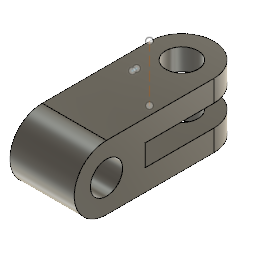
hinge1 (Autodesk Fusion 360 design; units mm, degrees)
Autodesk Fusion 360 part; units mm, degrees
note: some values were not read from the file. Set by a fixed rule: which sketch regions a step uses.
sketch "Sketch1" plane through (0, 0, 0) normal (1, 0, 0) x (0, 1, 0)
  line L0 (0, 0) -> (250, 0)
  line L1 (250, 0) -> (250, 150)
  line L2 (250, 150) -> (0, 150)
  line L3 (0, 150) -> (0, 0)
  circle A0 centre (0, 75) radius 75
  dimension "d1" = 250
  dimension "d2" = 150
  constraint coincident L0.start L3.end
  constraint horizontal L0
  constraint perpendicular L0 L1
  constraint perpendicular L1 L2
  constraint perpendicular L0 L3
  constraint coincident L2.end A0
  constraint tangent L2 A0
  constraint coincident L0.start A0
  measures "d1" distance of L0.start L0.end
  measures "d2" distance of L0.end L1.end
sketch "Sketch2" plane through (0, 0, 0) normal (1, 0, 0) x (0, 1, 0)
extrude "Extrude1" add sketch "Sketch1" along normal blind 150
sketch "Sketch3" plane through (0, 0, 0) normal (-1, 0, 0) x (0, -1, 0)
  line L0 (0, 150) -> (-250, 150)
  line L1 (-250, 150) -> (-250, 0)
  line L2 (-250, 0) -> (0, 0)
  arc A0 (0, 0) -> (0, 150) centre (0, 75) ccw
  line L3 (0, 150) -> (0, 0)
  circle A1 centre (0, 75) radius 37.5
  dimension "d5" = 75
  constraint coincident L0.start A0.end
  constraint coincident L2.end A0.start
  constraint concentric A0 A1
  measures "d5" diameter of A1
extrude "Extrude2" cut sketch "Sketch3" against normal blind 150 contours L3 A1 | L3 A1
sketch "Sketch4" plane through (150, 0, 0) normal (1, 0, 0) x (0, 1, 0)
  circle A0 centre (0, 75) radius 37.5
  line L0 (250, 150) -> (0, 150)
  arc A1 (0, 150) -> (0, 0) centre (0, 75) ccw
  line L1 (0, 0) -> (250, 0)
  line L2 (250, 0) -> (250, 150)
  line L3 (250, 150) -> (250, 0) construction
  line L4 (250, 75) -> (90, 75) construction
  line L5 (90, 75) -> (90, 100)
  line L6 (90, 75) -> (90, 50)
  line L7 (90, 100) -> (250, 100)
  line L8 (250, 50) -> (90, 50)
  dimension "d8" = 25
  dimension "d9" = 25
  constraint coincident L0.start L2.end
  constraint coincident L1.end L2.start
  constraint midpoint L2 L4.start
  constraint perpendicular L2 L4
  constraint perpendicular L0 L5
  constraint perpendicular L4 L6
  constraint coincident L2 L7.end
  constraint perpendicular L2 L7
  constraint coincident L2 L8.start
  constraint perpendicular L6 L8
  measures "d8" distance of L4.end L5.end
  measures "d9" distance of L4.end L6.end
extrude "Extrude3" cut sketch "Sketch4" against normal blind 150 contours L2 L5 L6 L7 L8
sketch "Sketch5" plane through (0, 0, 0) normal (0, 0, -1) x (1, 0, 0)
  line L0 (0, 0) -> (0, -250)
  line L1 (0, -250) -> (150, -250)
  line L2 (150, -250) -> (150, 0)
  line L3 (150, 0) -> (0, 0)
  line L4 (0, -250) -> (150, -250) construction
  circle A0 centre (75, -250) radius 75
  dimension "d12" = 150
  constraint coincident L0.end L1.start
  constraint coincident L1.end L2.start
  constraint midpoint L1 A0.centre
  measures "d12" diameter of A0
extrude "Extrude4" add sketch "Sketch5" against normal blind 50 contours L1 A0 picked at (76.8683, -274.9301)
sketch "Sketch6" plane through (0, 0, 0) normal (1, 0, 0) x (0, 1, 0)
  line L0 (220, 110) -> (210, 110)
  line L1 (250, 150) -> (250, 20) construction
  constraint horizontal L0
  constraint vertical L1
sketch "Sketch7" plane through (0, 0, 150) normal (0, 0, 1) x (-1, 0, 0)
  line L0 (0, -250) -> (0, 0)
  line L1 (0, 0) -> (-150, 0)
  line L2 (-150, 0) -> (-150, -250)
  line L3 (-150, -250) -> (0, -250)
  circle A0 centre (-75, -250) radius 75
  dimension "d15" = 150
  constraint midpoint L3 A0.centre
  measures "d15" diameter of A0
extrude "Extrude5" add sketch "Sketch7" against normal blind 50 contours L3 A0 picked at (-76.8683, -274.9301)
sketch "Sketch8" plane through (0, 0, 150) normal (0, 0, 1) x (-1, 0, 0)
  line L0 (0, -250) -> (0, 0)
  line L1 (0, 0) -> (-150, 0)
  line L2 (-150, 0) -> (-150, -250)
  arc A0 (-150, -250) -> (0, -250) centre (-75, -250) ccw
  circle A1 centre (-75.6677, -249.6068) radius 37.5
  dimension "d18" = 75
  measures "d18" diameter of A1
extrude "Extrude6" cut sketch "Sketch8" against normal blind 50 contours A1
sketch "Sketch9" plane through (0, 0, 0) normal (0, 0, -1) x (1, 0, 0)
  line L0 (0, 0) -> (0, -250)
  arc A0 (0, -250) -> (150, -250) centre (75, -250) ccw
  line L1 (150, -250) -> (150, 0)
  line L2 (150, 0) -> (0, 0)
  circle A1 centre (75, -250) radius 37.5
  line L3 (0, -250) -> (150, -250) construction
  dimension "d21" = 75
  constraint concentric A0 A1
  constraint coincident L0.end A0.start
  constraint coincident A0.end L1.start
  measures "d21" diameter of A1
extrude "Extrude7" cut sketch "Sketch9" against normal blind 50 contours A1
